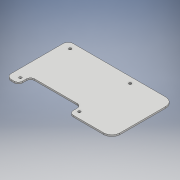
# Autodesk Inventor part: long_battery_mount
Saved by Autodesk Inventor 2017 (Build 210142000, 142)
## iProperties
Created: 2017-11-07
Part Number: long_battery_mount
Material: Generic
Document SubType Name: Modeling
Designer: Nic
Density: 1 g/cm^3
Appearance: Default
Author: Nic
Autodesk Inventor part; units mm, degrees
ref_plane "YZ Plane" through (0, 0, 0) normal (1, 0, 0) x (0, 1, 0)
ref_plane "XZ Plane" through (0, 0, 0) normal (0, 1, 0) x (-1, 0, 0)
ref_plane "XY Plane" through (0, 0, 0) normal (0, 0, 1) x (1, 0, 0)
sketch "Sketch1" plane through (0, 0, 0) normal (0, 0, 1) x (1, 0, 0)
  line L0 (96, -35) -> (96, 10)
  arc A0 (88, -43) -> (96, -35) centre (88, -35) ccw
  line L1 (54, -39) -> (54, -35)
  line L2 (50, -31) -> (8, -31)
  line L3 (4, -35) -> (4, -37.1118)
  line L4 (58, -43) -> (88, -43)
  arc A1 (8, -31) -> (4, -35) centre (8, -35) ccw
  arc A2 (54, -39) -> (58, -43) centre (58, -39) ccw
  arc A3 (54, -35) -> (50, -31) centre (50, -35) ccw
  line L5 (-34, 0) -> (96, 0) construction
  line L6 (88, 18) -> (-3, 18)
  circle A4 centre (59, 12) radius 1.3
  circle A5 centre (58, -37) radius 1.3
  line L7 (4, -37.1118) -> (4, -39)
  arc A6 (0, -43) -> (4, -39) centre (0, -39) ccw
  circle A7 centre (0, -37) radius 1.3
  line L8 (58, -37) -> (0, -37) construction
  line L9 (0, 0) -> (0, 18) construction
  line L10 (0, -43) -> (-3, -43)
  line L11 (-8, -38) -> (-8, 13)
  arc A8 (-3, 18) -> (-8, 13) centre (-3, 13) ccw
  arc A9 (-8, -38) -> (-3, -43) centre (-3, -38) ccw
  arc A10 (96, 10) -> (88, 18) centre (88, 10) ccw
  circle A11 centre (0, 12) radius 1.3
  point P0 (4, -43)
  point P1 (96, 18)
  point P2 (54, -31)
  point P3 (4, -31)
  dimension "d8" = 50
  dimension "d11" = 12
  dimension "d13" = 4
  dimension "d16" = 42
  dimension "d33" = 4
  dimension "d44" = 58
  dimension "d46" = 31
  dimension "d47" = 18
  dimension "d51" = 5
  dimension "d52" = 12
  dimension "d55" = 58
  dimension "d57" = 49
  dimension "d58" = 6
  dimension "d59" = 37
  dimension "d60" = 2.6
  dimension "d61" = 8
  dimension "d62" = 8
  dimension "d64" = 4
  constraints: 24 end point, 16 point on circle, 16 tangent, 12 centre point, 11 point on line, 6 equal radius, 5 perpendicular, 3 vertical, 2 horizontal, 1 collinear, 1 horizontal alignment
  measures "d8" distance of point (54, -31) point (4, -31)
  measures "d11" distance between parallel lines of L4 L2
  measures "d13" radius of A2
  measures "d16" distance between parallel lines of L0 L1
  measures "d33" radius of A6
  measures "d44" horizontal distance of L9.start L8.start
  measures "d46" distance between parallel lines of L5 L2
  measures "d47" distance between parallel lines of L5 L6
  measures "d51" radius of A8
  measures "d52" distance between parallel lines of L7 L11
  measures "d55" distance of L8.start L8.end
  measures "d57" vertical distance of A4.centre L8.start
  measures "d58" distance from line of L6 A4.centre
  measures "d59" distance from line of L0 A4.centre
  measures "d60" diameter of A4
  measures "d61" radius of A0
  measures "d62" radius of A10
  measures "d64" distance from line of L3 L8.end
extrude "Extrusion1" add sketch "Sketch1" along normal blind 1.56
body "Solid1"
